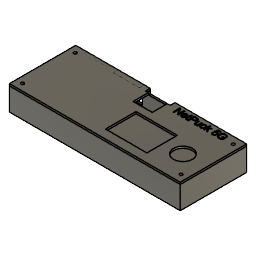
NetPuck5G (case without PCB) (Autodesk Fusion 360 design; units mm, degrees)
Autodesk Fusion 360 part; units mm, degrees
sketch "Sketch1" plane through (0, 0, 0) normal (0, 0, 1) x (1, 0, 0)
  line L0 (-28.4927, 28.0737) -> (151.5073, 28.0737)
  line L1 (151.5073, 28.0737) -> (151.5073, -41.9263)
  line L2 (151.5073, -41.9263) -> (-28.4927, -41.9263)
  line L3 (-28.4927, -41.9263) -> (-28.4927, 28.0737)
  dimension "d1" = 180
  dimension "d2" = 70
  constraint horizontal L0
  constraint vertical L1
  constraint horizontal L2
  constraint vertical L3
  measures "d1" distance of L0.start L0.end
  measures "d2" distance of L0.start L2.end
extrude "Extrude1" add sketch "Sketch1" along normal blind 15 makes body 1
extrude "Extrude4" add 1 faces at (31.5073, 4.7404, 15) along direction (0, 0, 1) blind 5 on bodies 1 bodies 1
extrude "Extrude10" add 1 faces at (31.5073, 4.7404, 0) along direction (0, 0, -1) blind 6 on bodies 1 bodies 1
shell "Shell2" thickness 2 removed faces 0 bodies 1
sketch "Sketch2" plane through (0, 0, 0) normal (0, 1, 0) x (1, 0, 0)
  line L0 (8.8279, -19.0645, 30) -> (-16.8627, -19.0645, 30)
  line L1 (-16.8627, -19.0645, 30) -> (-16.8627, -2.2174, 30)
  line L2 (-16.8627, -2.2174, 30) -> (8.8279, -2.2174, 30)
  line L3 (8.8279, -2.2174, 30) -> (8.8279, -19.0645, 30)
extrude "Extrude3" cut sketch "Sketch2" against normal blind 5 contours L0 L1 L2 L3 in plane through (0, 30, 0) normal (0, 1, 0) bodies 1
sketch "Sketch5" plane through (0, 28.0737, 0) normal (0, 1, 0) x (-1, 0, 0)
  line L0 (16.8627, 19.0645) -> (16.8627, 2.2174)
  line L1 (16.8627, 2.2174) -> (-8.8279, 2.2174)
  line L2 (-8.8279, 2.2174) -> (-8.8279, 19.0645)
  line L3 (-8.8279, 19.0645) -> (16.8627, 19.0645)
  line L4 (28.4927, -6) -> (28.4927, 20)
  line L5 (28.4927, 20) -> (-151.5073, 20)
  line L6 (-151.5073, 20) -> (-151.5073, -6)
  line L7 (-16.0496, 2.1977) -> (-43.5871, 2.1977)
  line L8 (-43.5871, 2.1977) -> (-43.5871, 19.1464)
  line L9 (-43.5871, 19.1464) -> (-16.0496, 19.1464)
  line L10 (-16.0496, 19.1464) -> (-16.0496, 2.1977)
  line L11 (-151.5073, -6) -> (28.4927, -6)
  constraint horizontal L7
  constraint vertical L8
  constraint horizontal L9
  constraint vertical L10
extrude "Extrude7" cut sketch "Sketch5" against normal blind 5 contours L7 L8 L9 L10 bodies 1
sketch "Sketch6" plane through (0, 28.0737, 0) normal (0, 1, 0) x (-1, 0, 0)
  line L0 (-82.1462, 2.5306) -> (-93.8005, 2.5306)
  line L1 (-93.8005, 2.5306) -> (-93.8005, 11.3546)
  line L2 (-93.8005, 11.3546) -> (-82.1462, 11.3546)
  line L3 (-82.1462, 11.3546) -> (-82.1462, 2.5306)
  constraint horizontal L0
  constraint vertical L1
  constraint horizontal L2
  constraint vertical L3
extrude "Extrude8" cut sketch "Sketch6" against normal blind 5 bodies 1
sketch "Sketch7" plane through (0, 28.0737, 0) normal (0, 1, 0) x (-1, 0, 0)
  line L0 (-76, 15) -> (-50, 15)
  line L1 (-50, 15) -> (-50, 20)
  line L2 (-50, 20) -> (-76, 20)
  line L3 (-76, 20) -> (-76, 15)
  constraint horizontal L0
  constraint vertical L1
  constraint horizontal L2
  constraint vertical L3
extrude "Extrude9" cut sketch "Sketch7" against normal blind 5 bodies 1
sketch "Sketch3" plane through (0, 0, 20) normal (0, 0, 1) x (-1, 0, 0)
  line L0 (28.4927, 41.9263) -> (-151.5073, 41.9263)
  line L1 (-151.5073, 41.9263) -> (-151.5073, -28.0737)
  line L2 (-50, -28.0737) -> (28.4927, -28.0737)
  line L3 (28.4927, -28.0737) -> (28.4927, 41.9263)
  line L4 (-73, -7) -> (-53, -7)
  line L5 (-53, -7) -> (-53, -29)
  line L6 (-53, -29) -> (-73, -29)
  line L7 (-73, -29) -> (-73, -7)
  line L8 (-76, -28.0737) -> (-76, -23.0737)
  line L9 (-76, -23.0737) -> (-50, -23.0737)
  line L10 (-50, -23.0737) -> (-50, -28.0737)
  line L11 (-151.5073, -28.0737) -> (-76, -28.0737)
  dimension "d13" = 20
  dimension "d14" = 22
  constraint horizontal L4
  constraint vertical L5
  constraint horizontal L6
  constraint vertical L7
  measures "d13" distance of L4.start L4.end
  measures "d14" distance of L4.start L6.end
extrude "Extrude5" cut sketch "Sketch3" against normal blind 5 contours L4 L5 L7 L9 bodies 1
sketch "Sketch4" plane through (0, 0, 20) normal (0, 0, 1) x (-1, 0, 0)
  line L0 (-73, -23.0737) -> (-73, -7)
  line L1 (-73, -7) -> (-53, -7)
  line L2 (-53, -7) -> (-53, -23.0737)
  line L3 (-50, -28.0737) -> (28.4927, -28.0737)
  line L4 (28.4927, -28.0737) -> (28.4927, 41.9263)
  line L5 (28.4927, 41.9263) -> (-151.5073, 41.9263)
  line L6 (-151.5073, 41.9263) -> (-151.5073, -28.0737)
  line L7 (-151.5073, -28.0737) -> (-76, -28.0737)
  line L8 (-63.6855, 0.6947) -> (-107.1741, 0.6947)
  line L9 (-107.1741, 0.6947) -> (-107.1741, 32.6958)
  line L10 (-107.1741, 32.6958) -> (-63.6855, 32.6958)
  line L11 (-63.6855, 32.6958) -> (-63.6855, 0.6947)
  line L12 (-53, -23.0737) -> (-50, -23.0737)
  line L13 (-50, -23.0737) -> (-50, -28.0737)
  line L14 (-76, -28.0737) -> (-76, -23.0737)
  line L15 (-76, -23.0737) -> (-73, -23.0737)
  constraint horizontal L8
  constraint vertical L9
  constraint horizontal L10
  constraint vertical L11
extrude "Extrude6" cut sketch "Sketch4" against normal blind 5 contours L8 L9 L10 L11 bodies 1
hole "Hole2" at (105.1439, 28.0737, 6.6405) direction (0, -1, 0) diameter 10 depth 12 tip angle 118 bodies 1
hole "Hole3" at (127.0248, -14.5769, 20) direction (0, 0, -1) diameter 20 depth 5 tip angle 180 bodies 1
move_body "Move7" bodies 1 to x (1, 0, 0) y (0, 1, 0) z (0, 0, 1) at (0, 0, 6)
sketch "Sketch8" plane through (0, 0, 2) normal (0, 0, 1) x (1, 0, 0)
  circle A0 centre (-22.2427, 20.8237) radius 4
  line L0 (8.8279, 26.0737) -> (-16.8627, 26.0737)
  line L1 (-26.4927, 26.0737) -> (-26.4927, -39.9263)
  circle A1 centre (-22.2427, -34.6763) radius 4
  line L2 (-26.4927, -39.9263) -> (149.5073, -39.9263)
  circle A2 centre (145.2573, -34.6763) radius 4
  line L3 (149.5073, -39.9263) -> (149.5073, 26.0737)
  circle A3 centre (145.2573, 20.8237) radius 4
  line L4 (149.5073, 26.0737) -> (108.8471, 26.0737)
  line L5 (-26.4927, -39.9263) -> (149.5073, -39.9263)
  line L6 (149.5073, -39.9263) -> (149.5073, 26.0737)
  line L7 (149.5073, 26.0737) -> (-26.4927, 26.0737)
  line L8 (-26.4927, 26.0737) -> (-26.4927, -39.9263)
  dimension "d39" = 8
  dimension "d40" = 5.25
  dimension "d41" = 4.25
  dimension "d42" = 8
  dimension "d43" = 5.25
  dimension "d44" = 4.25
  dimension "d45" = 8
  dimension "d46" = 5.25
  dimension "d47" = 4.25
  dimension "d48" = 8
  dimension "d49" = 4.25
  dimension "d50" = 5.25
  measures "d39" diameter of A0
  measures "d40" distance of A0.centre L0
  measures "d41" distance of A0.centre L1
  measures "d42" diameter of A1
  measures "d43" distance of A1.centre L2
  measures "d44" distance of L1 A1.centre
  measures "d45" diameter of A2
  measures "d46" distance of L2 A2.centre
  measures "d47" distance of A2.centre L3
  measures "d48" diameter of A3
  measures "d49" distance of L3 A3.centre
  measures "d50" distance of A3.centre L4
extrude "Extrude11" add sketch "Sketch8" along normal blind 6 contours A0 | A1 | A2 | A3 bodies 1
hole "Hole5" at (-22.2427, 20.8237, 8) direction (0, 0, -1) diameter 4.2 depth 5.7 tip angle 110 bodies 1
hole "Hole6" at (-22.2427, -34.6763, 8) direction (0, 0, -1) diameter 4.2 depth 5.7 tip angle 110 bodies 1
hole "Hole7" at (145.2573, 20.8237, 8) direction (0, 0, -1) diameter 4.2 depth 5.7 tip angle 110 bodies 1
hole "Hole8" at (145.2573, -34.6763, 8) direction (0, 0, -1) diameter 4.2 depth 5.7 tip angle 110 bodies 1
fillet "Fillet1" radius 2 4 edges at (-25.972, -33.2298, 2) (-25.972, 22.2702, 2) (141.528, 22.2702, 2) (141.528, -33.2298, 2) on bodies 1
sketch "Sketch9" plane through (0, 0, 26) normal (0, 0, 1) x (-1, 0, 0)
  circle A0 centre (-127.0248, 14.5769) radius 10
  line L0 (-107.1741, 0.6947) -> (-107.1741, 32.6958)
  line L1 (-107.1741, 32.6958) -> (-63.6855, 32.6958)
  line L2 (-63.6855, 32.6958) -> (-63.6855, 0.6947)
  line L3 (-63.6855, 0.6947) -> (-107.1741, 0.6947)
  line L4 (-73, -23.0737) -> (-73, -7)
  line L5 (-73, -7) -> (-53, -7)
  line L6 (-53, -7) -> (-53, -23.0737)
  line L7 (-53, -23.0737) -> (-50, -23.0737)
  line L8 (-50, -23.0737) -> (-50, -28.0737)
  line L9 (-50, -28.0737) -> (28.4927, -28.0737)
  line L10 (28.4927, -28.0737) -> (28.4927, 41.9263)
  line L11 (28.4927, 41.9263) -> (-151.5073, 41.9263)
  line L12 (-151.5073, 41.9263) -> (-151.5073, -28.0737)
  line L13 (-151.5073, -28.0737) -> (-76, -28.0737)
  line L14 (-76, -28.0737) -> (-76, -23.0737)
  line L15 (-76, -23.0737) -> (-73, -23.0737)
  line L16 (-77.1474, -17.1662) -> (-141.3157, -17.1745) construction
  line L17 (-141.3157, -17.1745) -> (-141.3144, -27.0505) construction
  line L18 (-141.3144, -27.0505) -> (-77.1462, -27.0423) construction
  line L19 (-77.1462, -27.0423) -> (-77.1474, -17.1662) construction
  dimension "d67" = 7
  dimension "d68" = 0
  text T0 "NetPuck 5G" font "Arial" height 7 align centre middle in box 64.1683 x 9.876 at (-77.1474, -17.1662) x (-1, -0.000129) y (0.000129, -1) spacing 1 kerned
emboss "Emboss1" depth -1 profiles "Sketch9" section 1 text T0 onto face at (-1.3285, -2.2842, 26) on bodies 1 bodies 1
sketch "Sketch15" plane through (0, 0, 26) normal (0, 0, 1) x (-1, 0, 0)
  spline S0 degree 3 poles (-97.1556, -19.4042) (-97.1966, -19.3862) (-97.2898, -19.3452) (-97.392, -19.3433) (-97.4492, -19.3422) knots 0 0 0 0 0.013315 0.030277 0.030277 0.030277 0.030277
  spline S1 degree 3 poles (-97.4492, -19.3422) (-97.5046, -19.3442) (-97.6309, -19.3487) (-97.7561, -19.3659) (-97.8264, -19.3757) knots 0 0 0 0 0.016614 0.037891 0.037891 0.037891 0.037891
  line L0 (-97.8264, -19.3757) -> (-97.9507, -18.6165)
  spline S2 degree 3 poles (-97.9507, -18.6165) (-97.8365, -18.5942) (-97.6219, -18.5524) (-97.4035, -18.5439) (-97.3013, -18.54) knots 0 0 0 0 0.034853 0.065473 0.065473 0.065473 0.065473
  spline S3 degree 3 poles (-97.3013, -18.54) (-97.1607, -18.5427) (-96.909, -18.5475) (-96.6777, -18.6449) (-96.5755, -18.6879) knots 0 0 0 0 0.041706 0.074669 0.074669 0.074669 0.074669
  spline S4 degree 3 poles (-96.5755, -18.6879) (-96.4966, -18.7397) (-96.3437, -18.84) (-96.2553, -18.9998) (-96.2126, -19.077) knots 0 0 0 0 0.027855 0.053928 0.053928 0.053928 0.053928
  spline S5 degree 3 poles (-96.2126, -19.077) (-96.1824, -19.2013) (-96.1015, -19.5338) (-96.1051, -19.8768) (-96.1074, -20.0917) knots 0 0 0 0 0.038244 0.102341 0.102341 0.102341 0.102341
  line L1 (-96.1074, -20.0917) -> (-96.107, -23.0091)
  line L2 (-96.107, -23.0091) -> (-95.4767, -23.009)
  line L3 (-95.4767, -23.009) -> (-95.4766, -23.6775)
  line L4 (-95.4766, -23.6775) -> (-96.1069, -23.6776)
  line L5 (-96.1069, -23.6776) -> (-96.1068, -24.9334)
  line L6 (-96.1068, -24.9334) -> (-96.9614, -25.4492)
  line L7 (-96.9614, -25.4492) -> (-96.9616, -23.6777)
  line L8 (-96.9616, -23.6777) -> (-97.8259, -23.6778)
  line L9 (-97.8259, -23.6778) -> (-97.826, -23.0094)
  line L10 (-97.826, -23.0094) -> (-96.9617, -23.0092)
  line L11 (-96.9617, -23.0092) -> (-96.9621, -20.044)
  spline S6 degree 3 poles (-96.9621, -20.044) (-96.9609, -19.9428) (-96.9589, -19.7832) (-96.9945, -19.628) (-97.0075, -19.5713) knots 0 0 0 0 0.030222 0.047628 0.047628 0.047628 0.047628
  spline S7 degree 3 poles (-97.0075, -19.5713) (-97.0253, -19.538) (-97.0612, -19.4704) (-97.1238, -19.4265) (-97.1556, -19.4042) knots 0 0 0 0 0.01116 0.022609 0.022609 0.022609 0.022609
  line L12 (-134.0058, -20.0536) -> (-134.0056, -21.3571)
  line L13 (-134.0056, -21.3571) -> (-131.9476, -21.3569)
  line L14 (-131.9476, -21.3569) -> (-131.9475, -22.1781)
  line L15 (-131.9475, -22.1781) -> (-134.9127, -22.1833)
  line L16 (-134.9127, -22.1833) -> (-134.9131, -19.5858)
  spline S8 degree 3 poles (-134.9131, -19.5858) (-134.6875, -19.417) (-134.2496, -19.0893) (-133.7479, -18.8721) (-133.5046, -18.7667) knots 0 0 0 0 0.084169 0.163431 0.163431 0.163431 0.163431
  spline S9 degree 3 poles (-133.5046, -18.7667) (-133.2616, -18.6866) (-132.7775, -18.527) (-132.2684, -18.5036) (-132.0148, -18.4919) knots 0 0 0 0 0.076362 0.152118 0.152118 0.152118 0.152118
  spline S10 degree 3 poles (-132.0148, -18.4919) (-131.682, -18.5087) (-131.03, -18.5415) (-130.4329, -18.8046) (-130.1406, -18.9334) knots 0 0 0 0 0.09904 0.193997 0.193997 0.193997 0.193997
  spline S11 degree 3 poles (-130.1406, -18.9334) (-129.8771, -19.0965) (-129.3519, -19.4217) (-129.0289, -19.9481) (-128.8679, -20.2105) knots 0 0 0 0 0.091578 0.182542 0.182542 0.182542 0.182542
  spline S12 degree 3 poles (-128.8679, -20.2105) (-128.7426, -20.5012) (-128.4856, -21.0969) (-128.4541, -21.7453) (-128.438, -22.0774) knots 0 0 0 0 0.094144 0.192973 0.192973 0.192973 0.192973
  spline S13 degree 3 poles (-128.438, -22.0774) (-128.455, -22.4109) (-128.4888, -23.0712) (-128.7405, -23.6825) (-128.8651, -23.985) knots 0 0 0 0 0.099357 0.196758 0.196758 0.196758 0.196758
  spline S14 degree 3 poles (-128.8651, -23.985) (-129.0202, -24.2597) (-129.3241, -24.7979) (-129.8413, -25.1354) (-130.0944, -25.3007) knots 0 0 0 0 0.093118 0.182426 0.182426 0.182426 0.182426
  spline S15 degree 3 poles (-130.0944, -25.3007) (-130.3779, -25.426) (-130.9661, -25.6861) (-131.6091, -25.7155) (-131.9423, -25.7307) knots 0 0 0 0 0.092128 0.191195 0.191195 0.191195 0.191195
  spline S16 degree 3 poles (-131.9423, -25.7307) (-132.1854, -25.722) (-132.6549, -25.7052) (-133.1003, -25.5566) (-133.3151, -25.4849) knots 0 0 0 0 0.072541 0.140105 0.140105 0.140105 0.140105
  spline S17 degree 3 poles (-133.3151, -25.4849) (-133.5058, -25.3983) (-133.8715, -25.2323) (-134.146, -24.9398) (-134.2773, -24.7999) knots 0 0 0 0 0.062141 0.119142 0.119142 0.119142 0.119142
  spline S18 degree 3 poles (-134.2773, -24.7999) (-134.3883, -24.6353) (-134.6263, -24.2822) (-134.7444, -23.8726) (-134.8075, -23.654) knots 0 0 0 0 0.059186 0.126952 0.126952 0.126952 0.126952
  line L17 (-134.8075, -23.654) -> (-133.9719, -23.4247)
  spline S19 degree 3 poles (-133.9719, -23.4247) (-133.9205, -23.5874) (-133.8266, -23.885) (-133.6571, -24.1465) (-133.5803, -24.265) knots 0 0 0 0 0.050912 0.093086 0.093086 0.093086 0.093086
  spline S20 degree 3 poles (-133.5803, -24.265) (-133.4904, -24.3632) (-133.3005, -24.5707) (-133.0458, -24.691) (-132.9117, -24.7543) knots 0 0 0 0 0.039551 0.083558 0.083558 0.083558 0.083558
  spline S21 degree 3 poles (-132.9117, -24.7543) (-132.7604, -24.8079) (-132.4484, -24.9184) (-132.1175, -24.9314) (-131.9471, -24.938) knots 0 0 0 0 0.047868 0.09869 0.09869 0.09869 0.09869
  spline S22 degree 3 poles (-131.9471, -24.938) (-131.7479, -24.9321) (-131.3721, -24.9209) (-131.0162, -24.8009) (-130.8489, -24.7445) knots 0 0 0 0 0.059406 0.112057 0.112057 0.112057 0.112057
  spline S23 degree 3 poles (-130.8489, -24.7445) (-130.7043, -24.6774) (-130.4271, -24.5488) (-130.207, -24.3371) (-130.1017, -24.2359) knots 0 0 0 0 0.047451 0.090949 0.090949 0.090949 0.090949
  spline S24 degree 3 poles (-130.1017, -24.2359) (-130.0126, -24.1288) (-129.8359, -23.9168) (-129.7184, -23.6671) (-129.6602, -23.5435) knots 0 0 0 0 0.041603 0.082422 0.082422 0.082422 0.082422
  spline S25 degree 3 poles (-129.6602, -23.5435) (-129.5822, -23.32) (-129.4231, -22.8639) (-129.4031, -22.3811) (-129.3929, -22.1348) knots 0 0 0 0 0.070593 0.144073 0.144073 0.144073 0.144073
  spline S26 degree 3 poles (-129.3929, -22.1348) (-129.4021, -21.8445) (-129.4191, -21.3031) (-129.6215, -20.8014) (-129.7154, -20.5687) knots 0 0 0 0 0.086325 0.161013 0.161013 0.161013 0.161013
  spline S27 degree 3 poles (-129.7154, -20.5687) (-129.8343, -20.3726) (-130.0702, -19.9833) (-130.4603, -19.7491) (-130.6538, -19.633) knots 0 0 0 0 0.067684 0.134314 0.134314 0.134314 0.134314
  spline S28 degree 3 poles (-130.6538, -19.633) (-130.8626, -19.5439) (-131.2808, -19.3653) (-131.7348, -19.3401) (-131.9622, -19.3275) knots 0 0 0 0 0.067516 0.135274 0.135274 0.135274 0.135274
  spline S29 degree 3 poles (-131.9622, -19.3275) (-132.1622, -19.3375) (-132.565, -19.3575) (-132.9453, -19.4917) (-133.1368, -19.5593) knots 0 0 0 0 0.059729 0.120288 0.120288 0.120288 0.120288
  spline S30 degree 3 poles (-133.1368, -19.5593) (-133.309, -19.6317) (-133.6187, -19.7619) (-133.8867, -19.9639) (-134.0058, -20.0536) knots 0 0 0 0 0.055772 0.100312 0.100312 0.100312 0.100312
  spline S31 degree 3 poles (-112.6621, -19.2009) (-112.8222, -19.2124) (-113.1342, -19.2348) (-113.3851, -19.4209) (-113.5072, -19.5114) knots 0 0 0 0 0.04708 0.09171 0.09171 0.09171 0.09171
  spline S32 degree 3 poles (-113.5072, -19.5114) (-113.6108, -19.6374) (-113.8397, -19.9155) (-113.9025, -20.2716) (-113.9368, -20.4664) knots 0 0 0 0 0.048154 0.106302 0.106302 0.106302 0.106302
  line L18 (-113.9368, -20.4664) -> (-114.782, -20.3567)
  spline S33 degree 3 poles (-114.782, -20.3567) (-114.7223, -20.0852) (-114.6079, -19.5648) (-114.2461, -19.175) (-114.0731, -18.9886) knots 0 0 0 0 0.081698 0.156599 0.156599 0.156599 0.156599
  spline S34 degree 3 poles (-114.0731, -18.9886) (-113.8686, -18.8445) (-113.4485, -18.5484) (-112.9352, -18.5126) (-112.6717, -18.4942) knots 0 0 0 0 0.073583 0.15115 0.15115 0.15115 0.15115
  spline S35 degree 3 poles (-112.6717, -18.4942) (-112.3454, -18.5187) (-111.7132, -18.5661) (-111.2312, -18.9761) (-110.998, -19.1744) knots 0 0 0 0 0.095415 0.184872 0.184872 0.184872 0.184872
  spline S36 degree 3 poles (-110.998, -19.1744) (-110.8138, -19.4414) (-110.4107, -20.0257) (-110.3812, -20.7381) (-110.3651, -21.1249) knots 0 0 0 0 0.095419 0.208798 0.208798 0.208798 0.208798
  spline S37 degree 3 poles (-110.3651, -21.1249) (-110.3739, -21.3842) (-110.3907, -21.8777) (-110.5578, -22.3419) (-110.6371, -22.5622) knots 0 0 0 0 0.077295 0.147077 0.147077 0.147077 0.147077
  spline S38 degree 3 poles (-110.6371, -22.5622) (-110.7381, -22.7538) (-110.9372, -23.1313) (-111.2912, -23.3691) (-111.4654, -23.4862) knots 0 0 0 0 0.063896 0.125837 0.125837 0.125837 0.125837
  spline S39 degree 3 poles (-111.4654, -23.4862) (-111.6557, -23.5761) (-112.0391, -23.7571) (-112.4625, -23.7819) (-112.6758, -23.7944) knots 0 0 0 0 0.0625 0.125938 0.125938 0.125938 0.125938
  spline S40 degree 3 poles (-112.6758, -23.7944) (-112.933, -23.7812) (-113.4201, -23.7564) (-113.8325, -23.4985) (-114.0272, -23.3767) knots 0 0 0 0 0.075808 0.143537 0.143537 0.143537 0.143537
  spline S41 degree 3 poles (-114.0272, -23.3767) (-114.1874, -23.2178) (-114.5221, -22.886) (-114.6394, -22.4286) (-114.7006, -22.1902) knots 0 0 0 0 0.066429 0.138714 0.138714 0.138714 0.138714
  line L19 (-114.7006, -22.1902) -> (-113.865, -22.0612)
  spline S42 degree 3 poles (-113.865, -22.0612) (-113.8218, -22.2172) (-113.7413, -22.5076) (-113.5369, -22.7279) (-113.4423, -22.8299) knots 0 0 0 0 0.04772 0.088865 0.088865 0.088865 0.088865
  spline S43 degree 3 poles (-113.4423, -22.8299) (-113.3345, -22.9051) (-113.1143, -23.0587) (-112.8462, -23.0779) (-112.7093, -23.0877) knots 0 0 0 0 0.038667 0.078996 0.078996 0.078996 0.078996
  spline S44 degree 3 poles (-112.7093, -23.0877) (-112.504, -23.0694) (-112.0992, -23.0333) (-111.8011, -22.7578) (-111.6541, -22.622) knots 0 0 0 0 0.05999 0.11828 0.11828 0.11828 0.11828
  spline S45 degree 3 poles (-111.6541, -22.622) (-111.5363, -22.4266) (-111.2649, -21.9765) (-111.2544, -21.4479) (-111.2485, -21.1489) knots 0 0 0 0 0.067373 0.155163 0.155163 0.155163 0.155163
  spline S46 degree 3 poles (-111.2485, -21.1489) (-111.2535, -20.8468) (-111.2624, -20.3166) (-111.5265, -19.8603) (-111.6402, -19.6639) knots 0 0 0 0 0.088758 0.155813 0.155813 0.155813 0.155813
  spline S47 degree 3 poles (-111.6402, -19.6639) (-111.7818, -19.5289) (-112.0682, -19.2557) (-112.4627, -19.2193) (-112.6621, -19.2009) knots 0 0 0 0 0.056945 0.115168 0.115168 0.115168 0.115168
  spline S48 degree 3 poles (-125.1342, -18.491) (-124.8357, -18.5088) (-124.2652, -18.5429) (-123.7979, -18.8698) (-123.5751, -19.0256) knots 0 0 0 0 0.087749 0.167712 0.167712 0.167712 0.167712
  spline S49 degree 3 poles (-123.5751, -19.0256) (-123.395, -19.2221) (-123.025, -19.6258) (-122.9325, -20.1663) (-122.885, -20.4437) knots 0 0 0 0 0.078227 0.160713 0.160713 0.160713 0.160713
  line L20 (-122.885, -20.4437) -> (-123.7874, -20.5202)
  spline S50 degree 3 poles (-123.7874, -20.5202) (-123.8262, -20.3197) (-123.8981, -19.9488) (-124.1413, -19.6615) (-124.2531, -19.5295) knots 0 0 0 0 0.060071 0.11111 0.11111 0.11111 0.11111
  spline S51 degree 3 poles (-124.2531, -19.5295) (-124.3822, -19.4327) (-124.6435, -19.2368) (-124.9692, -19.2109) (-125.1341, -19.1977) knots 0 0 0 0 0.047357 0.09588 0.09588 0.09588 0.09588
  spline S52 degree 3 poles (-125.1341, -19.1977) (-125.3335, -19.2178) (-125.735, -19.2581) (-126.034, -19.5293) (-126.1845, -19.6658) knots 0 0 0 0 0.05848 0.11774 0.11774 0.11774 0.11774
  spline S53 degree 3 poles (-126.1845, -19.6658) (-126.3097, -19.8409) (-126.5746, -20.2112) (-126.6005, -20.667) (-126.6141, -20.9073) knots 0 0 0 0 0.06326 0.133797 0.133797 0.133797 0.133797
  spline S54 degree 3 poles (-126.6141, -20.9073) (-126.6014, -21.1346) (-126.5774, -21.5634) (-126.3213, -21.9064) (-126.2009, -22.0676) knots 0 0 0 0 0.06658 0.125616 0.125616 0.125616 0.125616
  spline S55 degree 3 poles (-126.2009, -22.0676) (-126.049, -22.1915) (-125.7346, -22.448) (-125.329, -22.4773) (-125.1194, -22.4924) knots 0 0 0 0 0.05736 0.118748 0.118748 0.118748 0.118748
  spline S56 degree 3 poles (-125.1194, -22.4924) (-124.9855, -22.4852) (-124.7232, -22.4711) (-124.4859, -22.3587) (-124.3697, -22.3037) knots 0 0 0 0 0.039792 0.077964 0.077964 0.077964 0.077964
  spline S57 degree 3 poles (-124.3697, -22.3037) (-124.2649, -22.2372) (-124.0593, -22.1066) (-123.9152, -21.9104) (-123.8446, -21.8142) knots 0 0 0 0 0.036879 0.072353 0.072353 0.072353 0.072353
  line L21 (-123.8446, -21.8142) -> (-123.0376, -21.9192)
  line L22 (-123.0376, -21.9192) -> (-123.7151, -25.5147)
  line L23 (-123.7151, -25.5147) -> (-127.1961, -25.5152)
  line L24 (-127.1961, -25.5152) -> (-127.1962, -24.6939)
  line L25 (-127.1962, -24.6939) -> (-124.4028, -24.6935)
  line L26 (-124.4028, -24.6935) -> (-124.0259, -22.8122)
  spline S58 degree 3 poles (-124.0259, -22.8122) (-124.2351, -22.9403) (-124.6423, -23.1896) (-125.1175, -23.2314) (-125.3485, -23.2516) knots 0 0 0 0 0.072499 0.141068 0.141068 0.141068 0.141068
  spline S59 degree 3 poles (-125.3485, -23.2516) (-125.6414, -23.226) (-126.2233, -23.1749) (-126.6725, -22.802) (-126.8956, -22.6168) knots 0 0 0 0 0.085994 0.17082 0.17082 0.17082 0.17082
  spline S60 degree 3 poles (-126.8956, -22.6168) (-127.0794, -22.3852) (-127.4587, -21.9074) (-127.5032, -21.2979) (-127.5261, -20.9839) knots 0 0 0 0 0.086615 0.178696 0.178696 0.178696 0.178696
  spline S61 degree 3 poles (-127.5261, -20.9839) (-127.5048, -20.6801) (-127.4631, -20.0839) (-127.1339, -19.5856) (-126.9724, -19.3412) knots 0 0 0 0 0.08965 0.175984 0.175984 0.175984 0.175984
  spline S62 degree 3 poles (-126.9724, -19.3412) (-126.7236, -19.0933) (-126.2154, -18.5869) (-125.4996, -18.5234) (-125.1342, -18.491) knots 0 0 0 0 0.101995 0.208351 0.208351 0.208351 0.208351
  line L27 (-84.437, -24.1059) -> (-84.4377, -18.6052)
  line L28 (-84.4377, -18.6052) -> (-83.5496, -18.6051)
  line L29 (-83.5496, -18.6051) -> (-83.5487, -25.6051)
  line L30 (-83.5487, -25.6051) -> (-84.4989, -25.6052)
  line L31 (-84.4989, -25.6052) -> (-88.1763, -20.1097)
  line L32 (-88.1763, -20.1097) -> (-88.1756, -25.6057)
  line L33 (-88.1756, -25.6057) -> (-89.0637, -25.6058)
  line L34 (-89.0637, -25.6058) -> (-89.0646, -18.6058)
  line L35 (-89.0646, -18.6058) -> (-88.1144, -18.6056)
  line L36 (-88.1144, -18.6056) -> (-84.437, -24.1059)
  line L37 (-116.3815, -20.6195) -> (-116.3818, -18.6093)
  line L38 (-116.3818, -18.6093) -> (-115.5223, -18.6092)
  line L39 (-115.5223, -18.6092) -> (-115.5214, -25.6092)
  line L40 (-115.5214, -25.6092) -> (-116.3809, -25.6093)
  line L41 (-116.3809, -25.6093) -> (-116.3814, -21.6175)
  line L42 (-116.3814, -21.6175) -> (-118.4153, -23.6805)
  line L43 (-118.4153, -23.6805) -> (-119.5278, -23.6806)
  line L44 (-119.5278, -23.6806) -> (-117.5894, -21.7991)
  line L45 (-117.5894, -21.7991) -> (-119.7242, -18.6097)
  line L46 (-119.7242, -18.6097) -> (-118.6642, -18.6096)
  line L47 (-118.6642, -18.6096) -> (-116.9879, -21.2021)
  line L48 (-116.9879, -21.2021) -> (-116.3815, -20.6195)
  line L49 (-109.2809, -23.6793) -> (-109.2815, -18.6084)
  line L50 (-109.2815, -18.6084) -> (-108.5128, -18.6083)
  line L51 (-108.5128, -18.6083) -> (-108.5127, -19.3532)
  spline S63 degree 3 poles (-108.5127, -19.3532) (-108.299, -19.1025) (-107.8748, -18.6049) (-107.2257, -18.5304) (-106.9036, -18.4935) knots 0 0 0 0 0.095036 0.188617 0.188617 0.188617 0.188617
  spline S64 degree 3 poles (-106.9036, -18.4935) (-106.7574, -18.5002) (-106.469, -18.5135) (-106.1988, -18.6151) (-106.0656, -18.6653) knots 0 0 0 0 0.043604 0.086019 0.086019 0.086019 0.086019
  spline S65 degree 3 poles (-106.0656, -18.6653) (-105.947, -18.7226) (-105.726, -18.8294) (-105.5632, -19.0125) (-105.4878, -19.0973) knots 0 0 0 0 0.039059 0.07278 0.07278 0.07278 0.07278
  spline S66 degree 3 poles (-105.4878, -19.0973) (-105.4291, -19.1916) (-105.3059, -19.3894) (-105.2513, -19.6161) (-105.2227, -19.7347) knots 0 0 0 0 0.033102 0.069433 0.069433 0.069433 0.069433
  spline S67 degree 3 poles (-105.2227, -19.7347) (-105.2075, -19.8436) (-105.1704, -20.1095) (-105.1702, -20.3782) (-105.1701, -20.5369) knots 0 0 0 0 0.032944 0.080473 0.080473 0.080473 0.080473
  line L52 (-105.1701, -20.5369) -> (-105.1697, -23.6788)
  line L53 (-105.1697, -23.6788) -> (-106.0292, -23.6789)
  line L54 (-106.0292, -23.6789) -> (-106.0295, -20.8665)
  spline S68 degree 3 poles (-106.0295, -20.8665) (-106.0287, -20.6783) (-106.0273, -20.3746) (-106.067, -20.0737) (-106.0822, -19.9593) knots 0 0 0 0 0.056359 0.090963 0.090963 0.090963 0.090963
  spline S69 degree 3 poles (-106.0822, -19.9593) (-106.116, -19.8529) (-106.1824, -19.6441) (-106.3458, -19.4984) (-106.426, -19.4269) knots 0 0 0 0 0.0328 0.064423 0.064423 0.064423 0.064423
  spline S70 degree 3 poles (-106.426, -19.4269) (-106.5215, -19.3705) (-106.7215, -19.2524) (-106.9539, -19.2401) (-107.0754, -19.2336) knots 0 0 0 0 0.032752 0.068652 0.068652 0.068652 0.068652
  spline S71 degree 3 poles (-107.0754, -19.2336) (-107.2026, -19.242) (-107.4579, -19.2589) (-107.6865, -19.374) (-107.8012, -19.4319) knots 0 0 0 0 0.037809 0.075921 0.075921 0.075921 0.075921
  spline S72 degree 3 poles (-107.8012, -19.4319) (-107.9055, -19.5029) (-108.1108, -19.6427) (-108.2249, -19.8631) (-108.281, -19.9715) knots 0 0 0 0 0.037221 0.073226 0.073226 0.073226 0.073226
  spline S73 degree 3 poles (-108.281, -19.9715) (-108.3219, -20.1101) (-108.417, -20.4328) (-108.42, -20.7699) (-108.4217, -20.9623) knots 0 0 0 0 0.043153 0.100501 0.100501 0.100501 0.100501
  line L55 (-108.4217, -20.9623) -> (-108.4214, -23.6792)
  line L56 (-108.4214, -23.6792) -> (-109.2809, -23.6793)
  line L57 (-99.7027, -21.453) -> (-99.7031, -18.6071)
  line L58 (-99.7031, -18.6071) -> (-98.7768, -18.607)
  line L59 (-98.7768, -18.607) -> (-98.7758, -25.607)
  line L60 (-98.7758, -25.607) -> (-101.4164, -25.6074)
  spline S74 degree 3 poles (-101.4164, -25.6074) (-101.6216, -25.6067) (-101.978, -25.6057) (-102.3313, -25.56) (-102.4812, -25.5406) knots 0 0 0 0 0.061499 0.106781 0.106781 0.106781 0.106781
  spline S75 degree 3 poles (-102.4812, -25.5406) (-102.6426, -25.5079) (-102.9487, -25.4459) (-103.2181, -25.2882) (-103.3455, -25.2137) knots 0 0 0 0 0.049005 0.092972 0.092972 0.092972 0.092972
  spline S76 degree 3 poles (-103.3455, -25.2137) (-103.4571, -25.1229) (-103.6885, -24.9348) (-103.8322, -24.6734) (-103.9066, -24.5381) knots 0 0 0 0 0.042748 0.088562 0.088562 0.088562 0.088562
  spline S77 degree 3 poles (-103.9066, -24.5381) (-103.9686, -24.3881) (-104.095, -24.0823) (-104.111, -23.7516) (-104.1192, -23.5832) knots 0 0 0 0 0.048305 0.098484 0.098484 0.098484 0.098484
  spline S78 degree 3 poles (-104.1192, -23.5832) (-104.0972, -23.2988) (-104.054, -22.7395) (-103.7169, -22.2919) (-103.5512, -22.0718) knots 0 0 0 0 0.083642 0.164485 0.164485 0.164485 0.164485
  spline S79 degree 3 poles (-103.5512, -22.0718) (-103.2937, -21.8925) (-102.6831, -21.4673) (-101.9323, -21.4584) (-101.4981, -21.4532) knots 0 0 0 0 0.092246 0.218774 0.218774 0.218774 0.218774
  line L61 (-101.4981, -21.4532) -> (-99.7027, -21.453)
  spline S80 degree 3 poles (-92.6457, -19.1983) (-92.7955, -19.2072) (-93.085, -19.2244) (-93.3329, -19.3743) (-93.4526, -19.4467) knots 0 0 0 0 0.044247 0.085568 0.085568 0.085568 0.085568
  spline S81 degree 3 poles (-93.4526, -19.4467) (-93.5606, -19.5486) (-93.7969, -19.7718) (-93.9172, -20.0748) (-93.9825, -20.2394) knots 0 0 0 0 0.044006 0.096379 0.096379 0.096379 0.096379
  line L62 (-93.9825, -20.2394) -> (-94.8707, -20.1297)
  spline S82 degree 3 poles (-94.8707, -20.1297) (-94.7891, -19.8874) (-94.6313, -19.4184) (-94.2681, -19.0834) (-94.0925, -18.9216) knots 0 0 0 0 0.075332 0.145781 0.145781 0.145781 0.145781
  spline S83 degree 3 poles (-94.0925, -18.9216) (-93.8823, -18.7963) (-93.4361, -18.5304) (-92.9161, -18.505) (-92.641, -18.4916) knots 0 0 0 0 0.072283 0.153454 0.153454 0.153454 0.153454
  spline S84 degree 3 poles (-92.641, -18.4916) (-92.2949, -18.5145) (-91.633, -18.5583) (-91.1209, -18.9769) (-90.8766, -19.1766) knots 0 0 0 0 0.101196 0.193518 0.193518 0.193518 0.193518
  spline S85 degree 3 poles (-90.8766, -19.1766) (-90.6868, -19.4414) (-90.2766, -20.0134) (-90.2428, -20.7193) (-90.2246, -21.0984) knots 0 0 0 0 0.095729 0.206813 0.206813 0.206813 0.206813
  spline S86 degree 3 poles (-90.2246, -21.0984) (-90.2424, -21.4901) (-90.2755, -22.2172) (-90.6914, -22.811) (-90.8833, -23.0849) knots 0 0 0 0 0.11483 0.213147 0.213147 0.213147 0.213147
  spline S87 degree 3 poles (-90.8833, -23.0849) (-91.1232, -23.291) (-91.6147, -23.7132) (-92.2615, -23.7652) (-92.5926, -23.7918) knots 0 0 0 0 0.092396 0.189279 0.189279 0.189279 0.189279
  spline S88 degree 3 poles (-92.5926, -23.7918) (-92.9138, -23.7654) (-93.5432, -23.7137) (-94.0206, -23.3015) (-94.2543, -23.0996) knots 0 0 0 0 0.094002 0.184217 0.184217 0.184217 0.184217
  spline S89 degree 3 poles (-94.2543, -23.0996) (-94.4421, -22.8311) (-94.8494, -22.2487) (-94.8818, -21.5358) (-94.8992, -21.1515) knots 0 0 0 0 0.096332 0.208984 0.208984 0.208984 0.208984
  spline S90 degree 3 poles (-94.8992, -21.1515) (-94.8989, -21.1197) (-94.8982, -21.0433) (-94.8958, -20.9669) (-94.8945, -20.9223) knots 0 0 0 0 0.009551 0.022925 0.022925 0.022925 0.022925
  line L63 (-94.8945, -20.9223) -> (-91.1127, -20.9219)
  spline S91 degree 3 poles (-91.1127, -20.9219) (-91.1376, -20.6672) (-91.1835, -20.1975) (-91.4593, -19.8167) (-91.5856, -19.6422) knots 0 0 0 0 0.075127 0.138613 0.138613 0.138613 0.138613
  spline S92 degree 3 poles (-91.5856, -19.6422) (-91.737, -19.5127) (-92.0426, -19.2513) (-92.4434, -19.2161) (-92.6457, -19.1983) knots 0 0 0 0 0.058217 0.117519 0.117519 0.117519 0.117519
  circle A0 centre (-127.0248, 14.5769) radius 10
  line L64 (-107.1741, 0.6947) -> (-107.1741, 32.6958)
  line L65 (-107.1741, 32.6958) -> (-63.6855, 32.6958)
  line L66 (-63.6855, 32.6958) -> (-63.6855, 0.6947)
  line L67 (-63.6855, 0.6947) -> (-107.1741, 0.6947)
  line L68 (-73, -23.0737) -> (-73, -7)
  line L69 (-73, -7) -> (-53, -7)
  line L70 (-53, -7) -> (-53, -23.0737)
  line L71 (-53, -23.0737) -> (-50, -23.0737)
  line L72 (-50, -23.0737) -> (-50, -28.0737)
  line L73 (-50, -28.0737) -> (28.4927, -28.0737)
  line L74 (28.4927, -28.0737) -> (28.4927, 41.9263)
  line L75 (28.4927, 41.9263) -> (-151.5073, 41.9263)
  line L76 (-151.5073, 41.9263) -> (-151.5073, -28.0737)
  line L77 (-151.5073, -28.0737) -> (-76, -28.0737)
  line L78 (-76, -28.0737) -> (-76, -23.0737)
  line L79 (-76, -23.0737) -> (-73, -23.0737)
  circle A1 centre (21.75, -20.75) radius 1.5888
  circle A2 centre (21.75, 34.75) radius 1.589
  circle A3 centre (-144.75, 34.25) radius 1.5977
  circle A4 centre (-144.75, -20.75) radius 1.5986
hole "Hole12" at (144.75, 20.75, 26) at (144.75, -34.25, 26) at (-21.75, -34.75, 26) at (-21.75, 20.75, 26) direction (0, 0, -1) diameter 3.2 depth 1.9 tip angle 110 bodies 1
ref_plane "WorkPlane1" through (61.5073, -6.9263, 24) normal (0, 0, 1) x (1, 0, 0)
split "Split1" by plane through (61.5073, -6.9263, 24) normal (0, 0, 1) bodies 1 makes body 2 at (3.9824, -2.2858, 26)
equation "d68 = 'NetPuck 5G'"
